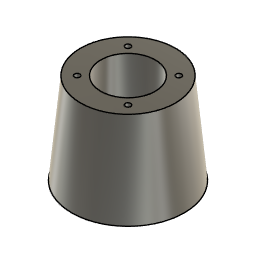
镭神N10P激光雷达固定座-可编辑 (Autodesk Fusion 360 design; units mm, degrees)
Autodesk Fusion 360 part; units mm, degrees
sketch "草图1" plane through (0, 0, 0) normal (0, 0, 1) x (1, 0, 0)
  circle A0 centre (0, 0) radius 26.15 construction
  circle A1 centre (0, 0) radius 25.5 construction
  circle A2 centre (0, 0) radius 31
  line L0 (0, 0) -> (46, 0) construction
  line L1 (0, 0) -> (0, 44.4165) construction
  line L2 (0, 0) -> (38.8757, 16.1028) construction
  circle A3 centre (23.5589, 9.7584) radius 2.35
  circle A4 centre (9.7584, 23.5589) radius 2.35
  circle A5 centre (-9.7584, 23.5589) radius 2.35
  circle A6 centre (-23.5589, 9.7584) radius 2.35
  circle A7 centre (-23.5589, -9.7584) radius 2.35
  circle A8 centre (-9.7584, -23.5589) radius 2.35
  circle A9 centre (9.7584, -23.5589) radius 2.35
  circle A10 centre (23.5589, -9.7584) radius 2.35
  dimension "d1" = 52.3
  dimension "d2" = 51
  dimension "d3" = 62
  dimension "d4" = 22.5
  dimension "d5" = 4.7
  dimension "d8" = 0
  dimension "d9" = 0
  dimension "d11" = 360
  constraint coincident A0.centre A1.centre
  constraint concentric A0 A2
  constraint horizontal L0
  constraint vertical L1
  constraint coincident A1 A3.centre
  constraint coincident L2 A3.centre
  measures "d1" diameter of A0
  measures "d2" diameter of A1
  measures "d3" diameter of A2
  measures "d4" angle of L0 L2
  measures "d5" diameter of A3
ref_plane "工作平面1" through (0, 0, 50) normal (0, 0, 1) x (1, 0, 0)
sketch "草图2" plane through (0, 0, 50) normal (0, 0, 1) x (1, 0, 0)
  circle A0 centre (0, 0) radius 26.15
  circle A1 centre (0, 0) radius 19.8 construction
  line L0 (0, 0) -> (28.4429, 28.4429) construction
  line L1 (0, 0) -> (40.2244, 0) construction
  circle A2 centre (14.0007, 14.0007) radius 1.5
  circle A3 centre (-14.0007, 14.0007) radius 1.5
  circle A4 centre (-14.0007, -14.0007) radius 1.5
  circle A5 centre (14.0007, -14.0007) radius 1.5
  circle A6 centre (14.0007, 14.0007) radius 1.5
  circle A7 centre (-14.0007, 14.0007) radius 1.5
  circle A8 centre (-14.0007, -14.0007) radius 1.5
  circle A9 centre (14.0007, -14.0007) radius 1.5
  dimension "d13" = 52.3
  dimension "d14" = 39.6
  dimension "d15" = 45
  dimension "d16" = 3
  dimension "d18" = 360
  dimension "d19" = 3
  constraint coincident A0.centre A1.centre
  constraint horizontal L1
  constraint coincident L0 A2.centre
  constraint coincident A1 A2.centre
  measures "d13" diameter of A0
  measures "d14" diameter of A1
  measures "d15" angle of L0 L1
  measures "d16" diameter of A2
  measures "d19" diameter of A6
loft "放样1" add profiles "草图1", "草图2" section 1 section 2
sketch "草图3" plane through (0, 0, 50) normal (0, 0, 1) x (-1, 0, 0)
  circle A0 centre (0, 0) radius 26.15
  line L0 (0, 0) -> (-33, 0) construction
  line L1 (0, 0) -> (0, -36) construction
  line L2 (0, 0) -> (-34.5137, -34.5137) construction
  circle A1 centre (0, 0) radius 19.8 construction
  circle A2 centre (-14.0007, -14.0007) radius 1.5
  circle A3 centre (14.0007, -14.0007) radius 1.5
  circle A4 centre (14.0007, 14.0007) radius 1.5
  circle A5 centre (-14.0007, 14.0007) radius 1.5
  dimension "d20" = 45
  dimension "d21" = 39.6
  dimension "d22" = 3
  dimension "d24" = 360
  constraint coincident A0.centre L0.start
  constraint horizontal L0
  constraint perpendicular L0 L1
  constraint coincident A1 A2.centre
  constraint coincident L2 A2.centre
  measures "d20" angle of L0 L2
  measures "d21" diameter of A1
  measures "d22" diameter of A2
hole "孔1" at (14.0007, 14.0007, 50) at (-14.0007, 14.0007, 50) at (-14.0007, -14.0007, 50) at (14.0007, -14.0007, 50) direction (0, 0, -1) diameter 3 depth 10 tip angle 118
sketch "草图4" plane through (0, 0, 0) normal (0, 0, -1) x (1, 0, 0)
  circle A0 centre (0, 0) radius 31
  line L0 (0, 0) -> (47.5733, 0) construction
  line L1 (0, 0) -> (0, -48.4854) construction
  line L2 (0, 0) -> (51.3087, -21.2528) construction
  circle A1 centre (0, 0) radius 25.5 construction
  circle A2 centre (23.5589, -9.7584) radius 2.35
  circle A3 centre (23.5589, 9.7584) radius 2.35
  circle A4 centre (9.7584, 23.5589) radius 2.35
  circle A5 centre (-9.7584, 23.5589) radius 2.35
  circle A6 centre (-23.5589, 9.7584) radius 2.35
  circle A7 centre (-23.5589, -9.7584) radius 2.35
  circle A8 centre (-9.7584, -23.5589) radius 2.35
  circle A9 centre (9.7584, -23.5589) radius 2.35
  dimension "d28" = 22.5
  dimension "d29" = 51
  dimension "d30" = 4.7
  dimension "d32" = 360
  constraint coincident A0.centre L0.start
  constraint horizontal L0
  constraint perpendicular L0 L1
  constraint coincident L2 A2.centre
  constraint coincident A1 A2.centre
  measures "d28" angle of L0 L2
  measures "d29" diameter of A1
  measures "d30" diameter of A2
hole "孔2" at (9.7584, -23.5589, 0) at (-9.7584, -23.5589, 0) at (-23.5589, -9.7584, 0) at (-23.5589, 9.7584, 0) at (-9.7584, 23.5589, 0) at (9.7584, 23.5589, 0) at (23.5589, 9.7584, 0) at (23.5589, -9.7584, 0) direction (0, 0, 1) diameter 4.7 depth 10 tip angle 180
hole "孔3" at (0, 0, 0) direction (0, 0, 1) diameter 30 end through all
